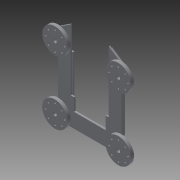
# Autodesk Inventor part: support_discovery
Saved by Autodesk Inventor 2014 SP1 (Build 180222100, 222)
## iProperties
Created: 2015-02-03
Part Number: support_discovery
Material: Générique
Document SubType Name: Modeling
Designer: astralien3000
Density: 1 g/cm^3
Appearance: Par défaut
Author: astralien3000
Autodesk Inventor part; units mm, degrees
ref_plane "YZ Plane" through (0, 0, 0) normal (1, 0, 0) x (0, 1, 0)
ref_plane "XZ Plane" through (0, 0, 0) normal (0, 1, 0) x (-1, 0, 0)
ref_plane "XY Plane" through (0, 0, 0) normal (0, 0, 1) x (1, 0, 0)
sketch "Esquisse1" plane through (0, 0, 0) normal (0, 1, 0) x (-1, 0, 0)
  line L0 (-60, 80) -> (60, 80)
  line L1 (60, 80) -> (60, -60)
  line L2 (60, -60) -> (-60, -60)
  line L3 (-60, -60) -> (-60, 80)
  circle A0 centre (50, 50) radius 3
  circle A1 centre (50, -50) radius 3
  circle A2 centre (-50, -50) radius 3
  circle A3 centre (-50, 50) radius 3
  point P0 (0, 0)
  dimension "d0" = 140
  dimension "d1" = 120
  dimension "d2" = 50
  dimension "d3" = 100
  dimension "d4" = 50
  dimension "d6" = 6
  dimension "d7" = 6
  dimension "d8" = 50
  dimension "d9" = 6
  dimension "d10" = 6
  dimension "d11" = 50
  dimension "d12" = 100
  dimension "d13" = 100
  dimension "d14" = 100
  dimension "d15" = 60
  dimension "d35" = 10
  constraints: 8 end point, 4 centre point, 2 parallel, 1 horizontal, 1 perpendicular
  measures "d0" distance of L2.end L0.start
  measures "d1" distance of L0.start L0.end
  measures "d2" horizontal distance of point (0, 0) A0.centre
  measures "d3" distance of A1.centre A0.centre
  measures "d4" horizontal distance of A0.centre point (0, 0)
  measures "d6" diameter of A0
  measures "d7" diameter of A1
  measures "d8" horizontal distance of A1.centre point (0, 0)
  measures "d9" diameter of A3
  measures "d10" diameter of A2
  measures "d11" horizontal distance of point (0, 0) A2.centre
  measures "d12" distance of A3.centre A2.centre
  measures "d13" distance of A3.centre A0.centre
  measures "d14" distance of A1.centre A2.centre
  measures "d15" distance from line of point (0, 0) L1
  measures "d35" distance from line of L2 A1.centre
extrude "Extrusion1" add sketch "Esquisse1" along normal blind 3
sketch "Esquisse2" plane through (0, 3, 0) normal (0, 1, 0) x (1, 0, 0)
  circle A0 centre (50, -50) radius 3 projected
  circle A1 centre (50, 50) radius 3 projected
  circle A2 centre (-50, 50) radius 3 projected
  circle A3 centre (-50, -50) radius 3 projected
  line L0 (-60, -80) -> (60, -80) projected
  line L1 (60, -80) -> (60, 60) projected
  line L2 (-60, 60) -> (-60, -80) projected
  line L3 (-40, -40) -> (-60, -40)
  line L4 (-60, -40) -> (-60, -60)
  line L5 (-60, -60) -> (-40, -60)
  line L6 (-40, -60) -> (-40, -40)
  line L7 (-60, 60) -> (-40, 60)
  line L8 (-40, 60) -> (-40, 40)
  line L9 (-40, 40) -> (-60, 40)
  line L10 (-60, 40) -> (-60, 60)
  line L11 (60, 60) -> (40, 60)
  line L12 (40, 60) -> (40, 40)
  line L13 (40, 40) -> (60, 40)
  line L14 (60, 40) -> (60, 60)
  line L15 (60, -40) -> (40, -40)
  line L16 (40, -40) -> (40, -60)
  line L17 (40, -60) -> (60, -60)
  line L18 (60, -60) -> (60, -40)
  line L19 (-60, 40) -> (-50, 40)
  line L20 (-50, 40) -> (-50, -40)
  line L21 (-50, -40) -> (-60, -40)
  line L22 (-60, -40) -> (-60, 40)
  line L23 (60, 40) -> (50, 40)
  line L24 (50, 40) -> (50, -40)
  line L25 (50, -40) -> (60, -40)
  line L26 (60, -40) -> (60, 40)
  line L27 (-30, -80) -> (30, -80)
  line L28 (30, -80) -> (30, 17)
  line L29 (30, 17) -> (-30, 17)
  line L30 (-30, 17) -> (-30, -80)
  line L31 (-60, -60) -> (-30, -80)
  line L32 (60, -60) -> (30, -80)
  line L33 (-40, 60) -> (40, 60)
  line L34 (-25, 17) -> (25, 17)
  line L35 (25, 17) -> (25, 37)
  line L36 (25, 37) -> (-25, 37)
  line L37 (-25, 37) -> (-25, 17)
  point P0 (0, 0)
  dimension "d19" = 20
  dimension "d20" = 20
  dimension "d21" = 20
  dimension "d22" = 20
  dimension "d23" = 20
  dimension "d24" = 20
  dimension "d25" = 20
  dimension "d26" = 20
  dimension "d27" = 10
  dimension "d28" = 10
  dimension "d29" = 10
  dimension "d30" = 10
  dimension "d31" = 60
  dimension "d32" = 97
  dimension "d33" = 120
  dimension "d34" = 30
  dimension "d36" = 5
  dimension "d37" = 5
  dimension "d38" = 20
  constraints: 70 end point, 16 parallel, 8 horizontal, 8 perpendicular, 6 point on line, 2 midpoint
  measures "d19" distance of L7.end L8.end
  measures "d20" distance of L7.start L7.end
  measures "d21" distance of L3.start L3.end
  measures "d22" distance of L5.end L3.start
  measures "d23" distance of L15.end L16.end
  measures "d24" distance of L16.end L17.end
  measures "d25" distance of L11.start L11.end
  measures "d26" distance of L11.end L12.end
  measures "d27" distance from line of L11 A1.centre
  measures "d28" distance from line of A2.centre L7
  measures "d29" distance from line of A3.centre L5
  measures "d30" distance from line of L17 A0.centre
  measures "d31" distance of L28.end L29.end
  measures "d32" distance of L27.end L28.end
  measures "d33" distance of L0.start L0.end
  measures "d34" distance between parallel lines of L2 L30
  measures "d36" distance between parallel lines of L28 L35
  measures "d37" distance between parallel lines of L30 L37
  measures "d38" distance between parallel lines of L36 L29
extrude "Extrusion2" cut sketch "Esquisse2" against normal through all contours L2 L31 L0 | L30 L29 L28 L0 | L32 L1 L0 | L2 L9 L20 L3 | L37 L36 L35 L29 | L15 L24 L13 L1
sketch "Esquisse3" plane through (0, 3, 0) normal (0, 1, 0) x (1, 0, 0)
  line L0 (60, -40) -> (50, -40) projected
  line L1 (50, -40) -> (50, 40) projected
  line L2 (-50, 40) -> (-50, -40) projected
  line L3 (-50, -40) -> (-60, -40) projected
  line L4 (-30, -80) -> (-30, 17) projected
  line L5 (-25, 37) -> (25, 37) projected
  line L6 (30, 17) -> (30, -80) projected
  line L7 (-50, 37) -> (-30, 37)
  line L8 (-30, 37) -> (-30, -40)
  line L9 (-30, -40) -> (-50, -40)
  line L10 (-50, -40) -> (-50, 37)
  line L11 (30, -40) -> (50, -40)
  line L12 (50, -40) -> (50, 37)
  line L13 (50, 37) -> (30, 37)
  line L14 (30, 37) -> (30, -40)
  point P0 (0, 0)
  constraints: 16 end point, 4 collinear, 4 parallel, 4 point on line, 2 horizontal, 2 perpendicular
extrude "Extrusion3" add sketch "Esquisse3" along normal blind 3
sketch "Esquisse5" plane through (-60, 0, 80) normal (0, 0, 1) x (1, 0, 0)
  line L0 (0, 3) -> (120, 3) projected
  line L1 (27.5, 2.25) -> (92.5, 2.25)
  line L2 (92.5, 2.25) -> (92.5, 3.75)
  line L3 (92.5, 3.75) -> (27.5, 3.75)
  line L4 (27.5, 3.75) -> (27.5, 2.25)
  point P0 (60, 0)
  dimension "d43" = 65
  dimension "d44" = 1.5
  dimension "d45" = 0.75
  dimension "d46" = 32.5
  constraints: 8 end point, 2 parallel, 1 horizontal, 1 perpendicular
  measures "d43" distance of L2.end L3.end
  measures "d44" distance between parallel lines of L1 L3
  measures "d45" distance between parallel lines of L0 L1
  measures "d46" distance from line of point (60, 0) L2
extrude "Extrusion4" cut sketch "Esquisse5" against normal blind 100
sketch "Esquisse6" plane through (0, 0, 0) normal (0, -1, 0) x (1, 0, 0)
  circle A0 centre (-50, 50) radius 3 projected
  circle A1 centre (-50, -50) radius 3 projected
  circle A2 centre (50, -50) radius 3 projected
  circle A3 centre (50, 50) radius 3 projected
  circle A4 centre (-50, 50) radius 20
  circle A5 centre (50, 50) radius 20
  circle A6 centre (50, -50) radius 20
  circle A7 centre (-50, -50) radius 20
  point P0 (0, 0)
  dimension "d49" = 40
  dimension "d50" = 40
  dimension "d51" = 40
  dimension "d52" = 40
  constraints: 4 centre point, 4 coincident
  measures "d49" diameter of A4
  measures "d50" diameter of A5
  measures "d51" diameter of A6
  measures "d52" diameter of A7
extrude "Extrusion5" add sketch "Esquisse6" along normal blind 5
sketch "Esquisse7" plane through (-50, -5, 50) normal (0, -1, 0) x (1, 0, 0)
  circle A0 centre (0, 0) radius 3 projected
  circle A1 centre (0, 0) radius 20 projected
  circle A2 centre (0, 0) radius 15 construction
  circle A3 centre (0, 15) radius 1.5
  line L0 (0, 0) -> (0, 20) construction
  circle A4 centre (-10.6066, 10.6066) radius 1.5
  circle A5 centre (-15, 0) radius 1.5
  circle A6 centre (-10.6066, -10.6066) radius 1.5
  circle A7 centre (0, -15) radius 1.5
  circle A8 centre (10.6066, -10.6066) radius 1.5
  circle A9 centre (15, 0) radius 1.5
  circle A10 centre (10.6066, 10.6066) radius 1.5
  point P0 (50, -50)
  dimension "d55" = 30
  dimension "d56" = 3
  dimension "d59" = 360
  constraints: 8 centre point, 2 end point, 2 vertical alignment, 1 coincident, 1 point on line, 1 vertical, 20 other
  measures "d56" diameter of A3
extrude "Extrusion6" cut sketch "Esquisse7" against normal through all contours A3 | A4 | A5 | A6 | A7 | A8 | A9 | A10
sketch "Esquisse8" plane through (50, -5, 50) normal (0, -1, 0) x (1, 0, 0)
  circle A0 centre (0, 0) radius 3
  circle A1 centre (0, 0) radius 20
  circle A2 centre (0, 0) radius 15 construction
  circle A3 centre (0, 15) radius 1.5
  line L0 (0, 0) -> (0, 20) construction
  circle A4 centre (-10.6066, 10.6066) radius 1.5
  circle A5 centre (-15, 0) radius 1.5
  circle A6 centre (-10.6066, -10.6066) radius 1.5
  circle A7 centre (0, -15) radius 1.5
  circle A8 centre (10.6066, -10.6066) radius 1.5
  circle A9 centre (15, 0) radius 1.5
  circle A10 centre (10.6066, 10.6066) radius 1.5
  point P0 (-50, -50)
  dimension "d65" = 30
  dimension "d66" = 3
  dimension "d67" = 360
  constraints: 9 centre point, 2 end point, 2 vertical alignment, 1 coincident, 1 point on line, 1 vertical, 21 other
  measures "d66" diameter of A3
extrude "Extrusion7" cut sketch "Esquisse8" against normal through all contours A3 | A4 | A5 | A6 | A7 | A8 | A9 | A10
sketch "Esquisse9" plane through (-50, -5, -50) normal (0, -1, 0) x (1, 0, 0)
  circle A0 centre (0, 0) radius 3
  circle A1 centre (0, 0) radius 20
  circle A2 centre (0, 0) radius 15 construction
  circle A3 centre (0, 15) radius 1.5
  line L0 (0, 0) -> (0, 20) construction
  circle A4 centre (-10.6066, 10.6066) radius 1.5
  circle A5 centre (-15, 0) radius 1.5
  circle A6 centre (-10.6066, -10.6066) radius 1.5
  circle A7 centre (0, -15) radius 1.5
  circle A8 centre (10.6066, -10.6066) radius 1.5
  circle A9 centre (15, 0) radius 1.5
  circle A10 centre (10.6066, 10.6066) radius 1.5
  point P0 (50, 50)
  dimension "d72" = 30
  dimension "d73" = 3
  dimension "d74" = 360
  constraints: 9 centre point, 2 end point, 2 vertical alignment, 1 coincident, 1 point on line, 1 vertical, 21 other
  measures "d73" diameter of A3
extrude "Extrusion8" cut sketch "Esquisse9" against normal through all contours A3 | A4 | A5 | A6 | A7 | A8 | A9 | A10
sketch "Esquisse10" plane through (50, -5, -50) normal (0, -1, 0) x (1, 0, 0)
  circle A0 centre (0, 0) radius 3
  circle A1 centre (0, 0) radius 20
  circle A2 centre (0, 0) radius 15 construction
  circle A3 centre (0, 15) radius 1.5
  line L0 (0, 0) -> (0, 20) construction
  circle A4 centre (-10.6066, 10.6066) radius 1.5
  circle A5 centre (-15, 0) radius 1.5
  circle A6 centre (-10.6066, -10.6066) radius 1.5
  circle A7 centre (0, -15) radius 1.5
  circle A8 centre (10.6066, -10.6066) radius 1.5
  circle A9 centre (15, 0) radius 1.5
  circle A10 centre (10.6066, 10.6066) radius 1.5
  point P0 (-50, 50)
  dimension "d79" = 30
  dimension "d80" = 3
  dimension "d81" = 360
  constraints: 9 centre point, 2 end point, 2 vertical alignment, 1 coincident, 1 point on line, 1 vertical, 21 other
  measures "d80" diameter of A3
extrude "Extrusion9" cut sketch "Esquisse10" against normal through all contours A3 | A4 | A5 | A6 | A7 | A8 | A9 | A10
equation "\"d15\" = 0.5 * d1"
equation "\"d27\" = 0.5 * d26"
equation "\"d28\" = 0.5 * d19"
equation "\"d29\" = 0.5 * d22"
equation "\"d30\" = 0.5 * d23"
equation "\"d34\" = -0.5 * d31 + 0.5 * d33"
equation "\"d45\" = 0.5 * d44"
equation "\"d46\" = 0.5 * d43"
